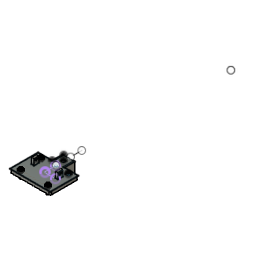
yCarriage (Autodesk Fusion 360 design; units mm, degrees)
Autodesk Fusion 360 part; units mm, degrees
note: some values were not read from the file. Chosen so that the rebuilt part matches the saved one: which sketch regions a step uses; that a step has no effect; which face or edge a step refers to.
sketch "Esquisse1" plane through (0, 0, 0) normal (0, 0, 1) x (1, 0, 0)
  line L0 (-40, -28) -> (-40, 28)
  line L1 (-40, 28) -> (-12, 28)
  line L2 (-12, 28) -> (-12, 49)
  line L3 (-12, 49) -> (12, 49)
  line L4 (12, 49) -> (12, 28)
  line L5 (12, 28) -> (40, 28)
  line L6 (40, 28) -> (40, -28)
  line L7 (40, -28) -> (-40, -28)
  circle A0 centre (-27.1, 21.1) radius 2.4
  circle A1 centre (-0.1034, 38.65) radius 2.9
  circle A2 centre (-27.1, -19.45) radius 2.4
  circle A3 centre (27.1, 21.1) radius 2.4
  circle A4 centre (27.1, -19.45) radius 2.4
  circle A5 centre (-0.0905, 23.6) radius 2.9
  line L8 (21.4, 11) -> (26.4, 11)
  line L9 (26.4, 11) -> (26.4, 1)
  line L10 (26.4, 1) -> (21.4, 1)
  line L11 (21.4, 1) -> (21.4, 11)
  line L12 (-21.4, 1) -> (-21.4, 11)
  line L13 (-26.4, 11) -> (-26.4, 1)
  line L14 (-26.4, 1) -> (-21.4, 1)
  line L15 (-21.4, 11) -> (-26.4, 11)
  circle A6 centre (27.1, 21.1) radius 3.3
  circle A7 centre (27.1, -19.45) radius 3.3
  circle A8 centre (-27.1, 21.1) radius 3.3
  circle A9 centre (-27.1, -19.45) radius 3.3
  line L16 (10, 362.4031) -> (10, 362.403)
  line L17 (10, 49) -> (10, 28)
  line L18 (10, 28) -> (12, 28)
  line L19 (0, 75) -> (0, 52.7229) construction
  line L20 (-10, 49) -> (-10, 28)
  line L21 (-10, 28) -> (-12, 28)
  line L22 (0, 1.75) -> (0, 22.5) construction
  line L23 (1.75, 0) -> (22.5, 0) construction
  dimension "d1" = 80
  dimension "d3" = 56
  dimension "d4" = 21
  dimension "d5" = 24
  dimension "d8" = 4.8
  dimension "d9" = 5.8
  dimension "d11" = 12.9
  dimension "d12" = 6.9
  dimension "d13" = 4.8
  dimension "d14" = 40.55
  dimension "d15" = 10.35
  dimension "d16" = 5.8
  dimension "d17" = 15.05
  dimension "d18" = 12.1034
  dimension "d19" = 54.2
  dimension "d20" = 5
  dimension "d21" = 10
  dimension "d22" = 13.6
  dimension "d23" = 17
  dimension "d27" = 6.6
  dimension "d28" = 12.9
  dimension "d29" = 6.9
  dimension "d30" = 6.6
  dimension "d31" = 6.6
  dimension "d32" = 6.6
  dimension "d33" = 2
  constraint vertical L0
  constraint perpendicular L0 L1
  constraint perpendicular L1 L2
  constraint perpendicular L2 L3
  constraint perpendicular L3 L4
  constraint perpendicular L4 L5
  constraint perpendicular L5 L6
  constraint perpendicular L0 L7
  constraint equal L0 L6
  constraint horizontal L8
  constraint vertical L9
  constraint horizontal L10
  constraint vertical L11
  constraint concentric A3 A6
  constraint coincident A4.centre A7.centre
  constraint coincident A0.centre A8.centre
  constraint coincident A2.centre A9.centre
  constraint perpendicular L3 L16
  constraint coincident L3 L17.start
  constraint perpendicular L3 L17
  constraint vertical L19
  constraint symmetric L4.end L19 L1.end
  constraint symmetric L17.start L19 L20.start
  constraint symmetric L17.end L19 L20.end
  constraint symmetric L0 L6 L22
  constraint symmetric L11 L12 L22
  constraint symmetric A2 A4 L22
  constraint symmetric L9 L13 L22
  constraint symmetric L10 L14 L22
  constraint symmetric L8 L15 L22
  constraint symmetric L17 L20 L22
  measures "d1" distance of L0 L6
  measures "d3" distance of L1 L7
  measures "d4" distance of L1.end L2.end
  measures "d5" distance of L2.end L3.end
  measures "d8" diameter of A0
  measures "d9" diameter of A1
  measures "d11" distance of L0 A0.centre
  measures "d12" distance of L1 A0.centre
  measures "d13" diameter of A2
  measures "d14" distance of A3.centre A4.centre
  measures "d15" distance of L3 A1.centre
  measures "d16" diameter of A5
  measures "d17" distance of A1.centre A5.centre
  measures "d18" distance of L4 A1.centre
  measures "d19" distance of A2.centre A4.centre
  measures "d20" distance of L8.start L8.end
  measures "d21" distance of L8.start L10.end
  measures "d22" distance of L6 L9
  measures "d23" distance of L5 L8
  measures "d27" diameter of A6
  measures "d28" distance of L6 A3.centre
  measures "d29" distance of L5 A3.centre
  measures "d30" diameter of A7
  measures "d31" diameter of A8
  measures "d32" diameter of A9
  measures "d33" distance of L4 L17
extrude "Extrusion2" add sketch "Esquisse1" against normal blind 6.4 contours L0 L1 L3 L5 L6 L7 L17 L18 L20 L21 | L8 L9 L10 L11 | L12 L13 L14 L15
extrude "Extrusion3" add sketch "Esquisse1" against normal blind 14.14 contours A6
extrude "Extrusion4" add sketch "Esquisse1" against normal blind 14.14 contours A8
extrude "Extrusion5" add sketch "Esquisse1" against normal blind 14.14 contours A7
extrude "Extrusion6" add sketch "Esquisse1" against normal blind 14.14 contours A9
extrude "Extrusion7" add sketch "Esquisse1" against normal blind 26.4 contours L2 L3 L20 L21 | L3 L4 L17 L18
extrude "Extrusion8" cut sketch "Esquisse1" against normal blind 20 contours A0 | A1 | A2 | A3 | A4 | A5
extrude "Extrusion9" add sketch "Esquisse1" along normal blind 12 contours L8 L9 L10 L11 | L12 L13 L14 L15
sketch "Esquisse2" plane through (26.4, 0, 0) normal (1, 0, 0) x (0, 1, 0)
  line L0 (1, 0) -> (11, 0)
  line L1 (11, 0) -> (11, 12)
  line L2 (11, 12) -> (1, 12)
  line L3 (1, 12) -> (1, 0)
  line L4 (8.84, 7.1) -> (3.16, 7.1)
  line L5 (3.16, 7.1) -> (3.16, 9.4)
  line L6 (3.16, 9.4) -> (8.84, 9.4)
  line L7 (8.84, 9.4) -> (8.84, 7.1)
  dimension "d53" = 2.6
  dimension "d54" = 2.3
  dimension "d55" = 2.16
  dimension "d56" = 2.16
  constraint horizontal L4
  constraint vertical L5
  constraint horizontal L6
  constraint vertical L7
  measures "d53" distance of L2 L6
  measures "d54" distance of L4 L6
  measures "d55" distance of L1 L7
  measures "d56" distance of L3 L5
extrude "Extrusion10" cut sketch "Esquisse2" against normal blind 90 contours L4 L5 L6 L7
sketch "Esquisse3" plane through (0, 0, 0) normal (0, 0, 1) x (1, 0, 0)
sketch "Esquisse4" plane through (0, 0, -20) normal (0, 0, 1) x (-1, 0, 0)
extrude "Extrusion11" [no effect]
fillet "Congé5" radius 0.8 1 edges at (-21.4, 6, 9.4)
fillet "Congé6" radius 0.8 1 edges at (26.4, 6, 9.4)
fillet "Congé7" radius 0.8 1 edges at (21.4, 6, 9.4)
fillet "Congé8" radius 0.8 1 edges at (-26.4, 6, 9.4)
chamfer "Chanfrein1" distance 0.8 angle 45 1 faces at (-24.3806, 19.2306, -8.98)
chamfer "Chanfrein2" distance 0.8 angle 45 1 faces at (-24.3806, -21.3194, -8.98)
chamfer "Chanfrein3" distance 0.8 angle 45 1 faces at (29.8194, 19.2306, -8.98)
chamfer "Chanfrein4" distance 0.8 angle 45 1 faces at (29.8194, -21.3194, -8.98)
fillet "Congé10" radius 2.5 1 edges at (-40, -28, -3.2)
fillet "Congé11" radius 2.5 1 edges at (40, -28, -3.2)
fillet "Congé12" radius 2.5 1 edges at (40, 28, -3.2)
fillet "Congé13" radius 2.5 1 edges at (-40, 28, -3.2)
